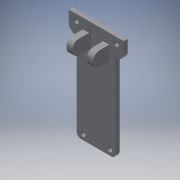
# Autodesk Inventor part: Part2
Saved by Autodesk Inventor 2016 (Build 200138000, 138)
## iProperties
Created: 2016-11-21
Part Number: Part2
Material: Generic
Document SubType Name: Modeling
Designer: Juraj
Density: 1 g/cm^3
Appearance: Default
Author: Juraj
Autodesk Inventor part; units mm, degrees
ref_plane "YZ Plane" through (0, 0, 0) normal (1, 0, 0) x (0, 1, 0)
ref_plane "XZ Plane" through (0, 0, 0) normal (0, 1, 0) x (-1, 0, 0)
ref_plane "XY Plane" through (0, 0, 0) normal (0, 0, 1) x (1, 0, 0)
sketch "Sketch1" plane through (0, 0, 0) normal (0, 1, 0) x (-1, 0, 0)
  line L0 (-6.9968, -12.4905) -> (-6.9968, 29.5095)
  line L1 (-6.9968, 29.5095) -> (-8.4968, 29.5095)
  line L2 (-7.9968, 46.0095) -> (-7.9968, 38.5095)
  line L3 (-7.9968, 38.5095) -> (-7.9968, 46.0095)
  arc A0 (-7.9968, 46.0095) -> (-9.4968, 47.5095) centre (-9.4968, 46.0095) ccw
  arc A1 (-7.9968, 46.0095) -> (-9.4968, 47.5095) centre (-9.4968, 46.0095) ccw
  line L4 (-9.4968, 47.5095) -> (-10.4968, 47.5095)
  line L5 (-9.4968, 47.5095) -> (-10.4968, 47.5095)
  line L6 (-11.9968, 46.0095) -> (-11.9968, 32.0095)
  arc A2 (-10.4968, 47.5095) -> (-11.9968, 46.0095) centre (-10.4968, 46.0095) ccw
  arc A3 (-11.9968, 32.0095) -> (-8.4968, 28.5095) centre (-8.4968, 32.0095) ccw
  line L7 (-11.9968, 46.0095) -> (-11.9968, 32.0095)
  arc A4 (-10.9968, 32.0095) -> (-8.4968, 29.5095) centre (-7.6108, 32.8955) ccw
  line L8 (-7.9968, 28.5095) -> (-7.9968, -12.4905)
  line L9 (-7.9968, 28.5095) -> (-8.4968, 28.5095)
  line L10 (-7.9968, 28.5095) -> (-8.4968, 28.5095)
  arc A5 (-11.9968, 32.0095) -> (-8.4968, 28.5095) centre (-8.4968, 32.0095) ccw
  line L11 (-8.4968, 28.5095) -> (-7.9968, 28.5095)
  line L12 (-7.9968, 28.5095) -> (-7.9968, -12.4905)
  arc A6 (-6.9968, -12.4905) -> (-5.8853, -13.4905) centre (-5.7634, -12.2372) ccw
  arc A7 (-7.9968, -12.4905) -> (-5.9968, -14.4905) centre (-5.9968, -12.4905) ccw
  arc A8 (-7.9968, -12.4905) -> (-5.9968, -14.4905) centre (-6.0394, -12.533) ccw
  line L13 (-5.9968, -14.4905) -> (1.5032, -14.4905)
  line L14 (1.5032, -14.4905) -> (1.5032, -16.2241)
  line L15 (-10.9968, 37.5095) -> (-10.9968, 32.0095)
  line L16 (-5.8853, -13.4905) -> (1.5032, -13.4905)
  line L17 (5.0532, -13.4905) -> (-2.0468, -13.4905)
  line L18 (-10.9968, 37.5095) -> (1.5032, 37.5095)
  line L19 (-7.9968, 38.5095) -> (1.5032, 38.5095)
  line L20 (10.0032, 29.5095) -> (11.5032, 29.5095)
  arc A9 (11.5032, 29.5095) -> (14.0032, 32.0095) centre (10.6172, 32.8955) ccw
  line L21 (14.0032, 37.5095) -> (14.0032, 32.0095)
  line L22 (14.0032, 37.5095) -> (1.5032, 37.5095)
  line L23 (11.0032, 38.5095) -> (1.5032, 38.5095)
  line L24 (11.0032, 38.5095) -> (11.0032, 46.0095)
  arc A10 (12.5032, 47.5095) -> (11.0032, 46.0095) centre (12.5032, 46.0095) ccw
  line L25 (12.5032, 47.5095) -> (13.5032, 47.5095)
  arc A11 (15.0032, 46.0095) -> (13.5032, 47.5095) centre (13.5032, 46.0095) ccw
  line L26 (15.0032, 46.0095) -> (15.0032, 32.0095)
  arc A12 (11.5032, 28.5095) -> (15.0032, 32.0095) centre (11.5032, 32.0095) ccw
  line L27 (11.0032, 28.5095) -> (11.5032, 28.5095)
  line L28 (11.0032, 28.5095) -> (11.0032, -12.4905)
  line L29 (10.0032, -12.4905) -> (10.0032, 29.5095)
  line L30 (8.8916, -13.4905) -> (1.5032, -13.4905)
  line L31 (9.0032, -14.4905) -> (1.5032, -14.4905)
  arc A13 (9.0032, -14.4905) -> (11.0032, -12.4905) centre (9.0032, -12.4905) ccw
  arc A14 (8.8916, -13.4905) -> (10.0032, -12.4905) centre (8.7697, -12.2372) ccw
  circle A15 centre (11.3532, 34.5095) radius 1.25
  circle A16 centre (11.3532, 34.5095) radius 1.25
  circle A17 centre (-8.3468, 34.5095) radius 1.25
  circle A18 centre (-8.3468, 34.5095) radius 1.25
  circle A19 centre (8.0032, -11.8434) radius 1.25
  circle A20 centre (8.0032, -11.8434) radius 1.25
  circle A21 centre (-4.9968, -11.8434) radius 1.25
  circle A22 centre (-4.9968, -11.8434) radius 1.25
  line L32 (-10.9968, 37.5095) -> (-11.9968, 37.5095)
  line L33 (14.0032, 37.5095) -> (15.0032, 37.5095)
  line L34 (15.0032, 37.5095) -> (15.0032, 46.0095)
  line L35 (-11.9968, 37.5095) -> (-11.9968, 46.0095)
  point P0 (0, 0)
  point P1 (5.0518, -13.4905)
  point P2 (-2.0454, -13.4905)
  point P3 (-2.0454, 37.5095)
  point P4 (5.0518, 37.5095)
  dimension "d11" = 2.5
  dimension "d6" = 3.5
  dimension "d7" = 1
  dimension "d8" = 1
  dimension "d9" = 3.5
  dimension "d10" = 0
  constraints: 72 end point, 30 point on circle, 22 centre point, 22 symmetric about line, 5 collinear, 4 coincident, 4 vertical, 3 point on line, 2 concentric, 2 tangent, 1 horizontal, 1 midpoint, 1 perpendicular, 9 other
  measures "d6" radius of A4
  measures "d7" distance between parallel lines of L8 L0
  measures "d8" distance between parallel lines of L9 L1
  measures "d9" radius of A3
  measures "d10" horizontal distance of L1.end L9.end
extrude "Extrusion1" add sketch "Sketch1" along normal blind 2 contours A6 L16 L17 L30 A14 L29 L20 A9 L21 L33 L26 A12 L27 L28 A13 L31 L13 A7 L8 L9 A3 L6 L32 L15 A4 L1 L0 | L0 L1 A4 L15 L18 L22 L21 A9 L20 L29 A14 L30 L17 L16 A6
sketch "Sketch2" plane through (0, 0, 0) normal (0, -1, 0) x (1, 0, 0)
  line L0 (4.9968, 25.5095) -> (1.9968, 25.5095)
  line L1 (1.9968, 25.5095) -> (1.9968, 32.5095)
  line L2 (1.9968, 32.5095) -> (4.9968, 32.5095)
  line L3 (4.9968, 32.5095) -> (4.9968, 25.5095)
  line L4 (-5.0032, 25.5095) -> (-8.0032, 25.5095)
  line L5 (-8.0032, 25.5095) -> (-8.0032, 32.5095)
  line L6 (-8.0032, 32.5095) -> (-5.0032, 32.5095)
  line L7 (-5.0032, 32.5095) -> (-5.0032, 25.5095)
  line L8 (-8.8916, -13.4905) -> (5.8853, -13.4905) projected
  line L9 (-15.0032, 37.5095) -> (11.9968, 37.5095) projected
  line L10 (-11.0032, -12.4905) -> (-11.0032, 28.5095) projected
  point P0 (0, 0)
  point P1 (10.9968, 37.5095)
  point P2 (-14.0032, 37.5095)
  dimension "d15" = 7
  dimension "d18" = 3
  dimension "d21" = 7
  dimension "d32" = 3
  dimension "d36" = 5
  dimension "d41" = 3
  constraints: 16 end point, 4 parallel, 2 horizontal, 2 perpendicular, 2 point on line
  measures "d15" distance between parallel lines of L1 L7
  measures "d18" distance of L1.end L2.end
  measures "d21" distance of L2.end L0.start
  measures "d32" distance of L5.end L6.end
  measures "d36" distance between parallel lines of L9 L2
  measures "d41" distance between parallel lines of L5 L10
extrude "Extrusion2" add sketch "Sketch2" along normal blind 8
fillet "Fillet1" radius 3 4 edges at (-6.5032, -8, 32.5095) (-6.5032, -8, 25.5095) (3.4968, -8, 32.5095) (3.4968, -8, 25.5095)
sketch "Sketch4" plane through (0, 0, 0) normal (0, -1, 0) x (1, 0, 0)
  line L0 (1.9968, 23.5095) -> (-5.0032, 23.5095)
  line L1 (-5.0032, 23.5095) -> (-5.0032, 34.5095)
  line L2 (-5.0032, 34.5095) -> (1.9968, 34.5095)
  line L3 (1.9968, 34.5095) -> (1.9968, 23.5095)
  line L4 (-5.0032, 32.5095) -> (-8.0032, 32.5095) projected
  line L5 (-5.0032, 25.5095) -> (-8.0032, 25.5095) projected
  point P0 (0, 0)
  dimension "d37" = 2
  dimension "d38" = 2
  constraints: 8 end point, 2 parallel, 1 horizontal, 1 perpendicular
  measures "d37" distance between parallel lines of L4 L2
  measures "d38" distance between parallel lines of L5 L0
extrude "Extrusion4" cut sketch "Sketch4" against normal blind 1
sketch "Sketch5" plane through (4.9968, 0, 32.5095) normal (1, 0, 0) x (0, 0, -1)
  circle A0 centre (3.5, -4.5) radius 1.5
  line L0 (4, 0) -> (45, 0) projected
  line L1 (7, 0) -> (7, -5) projected
  line L2 (0, 0) -> (0, -5) projected
  point P0 (32.5095, 0)
  dimension "d42" = 3
  dimension "d43" = 4.5
  dimension "d44" = 3.5
  dimension "d45" = 3.5
  constraints: 1 centre point
  measures "d42" diameter of A0
  measures "d43" distance from line of L0 A0.centre
  measures "d44" distance from line of L1 A0.centre
  measures "d45" distance from line of L2 A0.centre
extrude "Extrusion5" cut sketch "Sketch5" against normal blind 15
sketch "Sketch6" plane through (0, 0, 0) normal (0, -1, 0) x (1, 0, 0)
  line L0 (5.9968, -14.4905) -> (-9.0032, -14.4905) projected
  line L1 (-1.5032, -14.4905) -> (-1.5032, -0.2916)
  line L2 (-1.5032, -7.5767) -> (-6.5032, -7.5767)
  circle A0 centre (-6.5032, -7.5767) radius 1.5
  circle A1 centre (3.4968, -7.5767) radius 1.5
  point P0 (0, 0)
  dimension "d48" = 3
  dimension "d49" = 5
  constraints: 4 end point, 2 centre point, 1 coincident, 1 horizontal, 1 midpoint, 1 point on line, 1 symmetric about line, 1 vertical, 1 other
  measures "d48" diameter of A0
  measures "d49" distance of L2.start L2.end
extrude "Extrusion6" cut sketch "Sketch6" against normal blind 3
equation "\"d6\" = d9"
equation "\"d7\" = d12"
equation "\"d8\" = d12"
equation "\"d32\" = d18"
equation "\"d12\" = 1"
body "Solid1"
